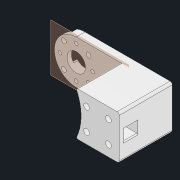
# Autodesk Inventor part: scara-base22
Saved by Autodesk Inventor 2022 (Build 260153000, 153)
## iProperties
Created: 2021-10-15
Part Number: scara-base22
Material: ABS プラスチック
Document SubType Name: Modeling
Designer: Yuta Kage
Density: 1.06 g/cm^3
Appearance: 滑らか - 白
Description: 印刷
Mass: 77.8231 g
Surface Area: 222.944 cm^2
Volume: 73.418 cm^3
Author: Yuta Kage
Autodesk Inventor part; units mm, degrees
ref_plane "YZ Plane" through (0, 0, 0) normal (1, 0, 0) x (0, 1, 0)
sketch "スケッチ1" plane through (0, 0, 0) normal (0, 0, 1) x (1, 0, 0)
  line L0 (0, -20) -> (80, -20)
  line L1 (80, -20) -> (80, 20)
  line L2 (80, 20) -> (0, 20)
  arc A0 (0, 20) -> (0, -20) centre (0, 0) ccw
  dimension "d0" = 40
  dimension "d2" = 40
  dimension "d51" = 80
  constraints: 6 end point, 2 point on circle, 1 centre point, 1 coincident, 1 horizontal, 1 parallel, 1 perpendicular
  measures "d0" distance of L0.end L1.end
  measures "d2" diameter of A0
  measures "d51" distance of L1.end L2.end
extrude "押し出し1" add sketch "スケッチ1" along normal blind 8
sketch "スケッチ2" plane through (0, 0, 8) normal (0, 0, 1) x (1, 0, 0)
  circle A0 centre (0, 0) radius 45
  line L0 (80, -20) -> (80, 20) projected
  line L1 (80, 20) -> (0, 20) projected
  line L2 (0, -20) -> (80, -20) projected
  arc A1 (0, 20) -> (0, -20) centre (0, 0) ccw projected
  point P0 (40.3113, 20)
  point P1 (40.3113, -20)
  point P2 (-40.3113, -20)
  point P3 (-40.3113, 20)
  dimension "d7" = 90
  constraints: 1 centre point, 1 coincident
  measures "d7" diameter of A0
extrude "押し出し2" add sketch "スケッチ2" along normal blind 40.5 contours A0 L1 L0 L2
sketch "スケッチ3" plane through (0, 0, 0) normal (0, 0, -1) x (-1, 0, 0)
  line L0 (-50, 10) -> (-70, 10)
  line L1 (-70, 10) -> (-70, -10)
  line L2 (-70, -10) -> (-50, -10)
  line L3 (-50, -10) -> (-50, 10)
  line L4 (-50, 10) -> (-70, -10) construction
  line L5 (-70, 10) -> (-50, -10) construction
  line L6 (-80, -20) -> (-80, 20) projected
  point P0 (-60, 0)
  point P1 (0, 0)
  dimension "d11" = 20
  dimension "d52" = 20
  dimension "d53" = 10
  constraints: 12 end point, 2 parallel, 1 horizontal, 1 horizontal alignment, 1 midpoint, 1 perpendicular
  measures "d11" distance of L1.end L0.end
  measures "d52" distance of L1.end L2.end
  measures "d53" distance between parallel lines of L6 L1
hole "穴1" at (50, -10, 0) at (50, 10, 0) at (70, -10, 0) at (70, 10, 0) direction (0, 0, 1) diameter 5.3 end through all clearance for "Socket Head Cap Screw" size "M5" standard "Ansi Metric M Profile"
sketch "スケッチ4" plane through (0, 0, 0) normal (0, 0, -1) x (-1, 0, 0)
  circle A0 centre (0, 0) radius 8.5
  dimension "d19" = 17
  constraints: 1 centre point, 1 coincident
  measures "d19" diameter of A0
extrude "押し出し3" cut sketch "スケッチ4" against normal blind 20
sketch "スケッチ5" plane through (0, 0, 0) normal (0, 0, -1) x (-1, 0, 0)
  circle A0 centre (0, 0) radius 15
  point P0 (0, -15)
  point P1 (15, 0)
  point P2 (0, 15)
  point P3 (-15, 0)
  dimension "d22" = 30
  dimension "d25" = 360
  constraints: 1 coincident, 1 vertical alignment, 7 other
hole "穴2" at (-15, 0, 0) at (0, 15, 0) at (0, -15, 0) at (15, 0, 0) direction (0, 0, 1) diameter 3.4 end through all clearance for "Socket Head Cap Screw" size "M3" standard "Ansi Metric M Profile"
sketch "スケッチ6" plane through (0, 0, 0) normal (0, 0, -1) x (-1, 0, 0)
  circle A0 centre (0, 0) radius 16
  point P0 (11.3137, -11.3137)
  point P1 (11.3137, 11.3137)
  point P2 (-11.3137, 11.3137)
  point P3 (-11.3137, -11.3137)
  dimension "d34" = 32
  dimension "d37" = 360
  constraints: 1 coincident, 1 horizontal alignment, 8 other
hole "穴3" at (-11.3137, -11.3137, 0) at (-11.3137, 11.3137, 0) at (11.3137, 11.3137, 0) at (11.3137, -11.3137, 0) direction (0, 0, 1) diameter 4.5 end through all counterbore diameter 8 counterbore depth 4 clearance for "Socket Head Cap Screw" size "M4" standard "Ansi Metric M Profile"
fillet "フィレット2" radius 2 2 edges at (80, -20, 24.25) (80, 20, 24.25)
fillet "フィレット5" radius 1 2 edges at (40.3113, 20, 28.25) (40.3113, -20, 28.25)
ref_plane "作業平面1" through (0, 0, 44.5) normal (0, 0, 1) x (1, 0, 0)
sketch "スケッチ7" plane through (0, 0, 44.5) normal (0, 0, 1) x (1, 0, 0)
  circle A0 centre (50, -10) radius 2.65 projected
  circle A1 centre (50, 10) radius 2.65 projected
  circle A2 centre (50, 10) radius 8
  circle A3 centre (50, -10) radius 2.65 projected
  circle A4 centre (50, -10) radius 9
  line L0 (43.755, -5) -> (80, -5)
  line L1 (80, -5) -> (80, 5)
  line L2 (80, 5) -> (43.755, 5)
  line L3 (43.755, 5) -> (43.755, -5)
  line L4 (43.755, -5) -> (80, 5) construction
  line L5 (80, -5) -> (43.755, 5) construction
  line L6 (80, -18) -> (80, 18) projected
  point P0 (0, 0)
  point P1 (61.8775, 0)
  point P2 (61.8775, 0)
  point P3 (43.755, -3.5193)
  point P4 (57.4833, -5)
  point P5 (56.245, 5)
  dimension "d59" = 16
  dimension "d64" = 18
  dimension "d65" = 10
  constraints: 12 end point, 3 midpoint, 2 coincident, 2 parallel, 1 centre point, 1 horizontal, 1 horizontal alignment, 1 perpendicular, 1 point on line, 3 other
  measures "d64" diameter of A4
  measures "d65" distance of L0.end L1.end
extrude "押し出し4" cut sketch "スケッチ7" against normal blind 13 contours A0 | A1 | A2 L2 | L2 A2 | A2 L2 L1 L0 A4 L3 | L3 L0 A4 | A4 L0 L3
sketch "スケッチ8" plane through (0, 0, 31.5) normal (0, 0, 1) x (1, 0, 0)
  circle A0 centre (50, 10) radius 5
  circle A1 centre (50, -10) radius 5
  circle A2 centre (50, -10) radius 2.65 projected
  circle A3 centre (50, 10) radius 2.65 projected
  point P0 (0, 0)
  dimension "d66" = 10
  dimension "d67" = 10
  constraints: 2 centre point, 2 coincident
  measures "d66" diameter of A0
  measures "d67" diameter of A1
extrude "押し出し5" add sketch "スケッチ8" along normal blind 0.5
sketch "スケッチ9" plane through (50, 10, 32) normal (0, 0, 1) x (1, 0, 0)
  circle A0 centre (0, -20) radius 5 projected
  circle A1 centre (0, 0) radius 5 projected
  circle A2 centre (0, -20) radius 3.95
  circle A3 centre (0, 0) radius 3.95
  circle A4 centre (0, -20) radius 2.65 projected
  circle A5 centre (0, 0) radius 2.65 projected
  point P0 (-50, -10)
  dimension "d70" = 7.9
  dimension "d71" = 7.9
  constraints: 2 centre point, 2 coincident
  measures "d70" diameter of A2
  measures "d71" diameter of A3
extrude "押し出し6" add sketch "スケッチ9" along normal blind 12 contours A2 | A3
sketch "スケッチ10" plane through (0, 0, 0) normal (0, 0, -1) x (-1, 0, 0)
  line L0 (50.5488, -20) -> (8, -20)
  line L1 (8, -20) -> (8, 20)
  line L2 (8, 20) -> (50.5488, 20)
  line L3 (50.5488, 20) -> (50.5488, -20)
  line L4 (50.5488, -20) -> (8, 20) construction
  line L5 (8, -20) -> (50.5488, 20) construction
  arc A0 (0, -20) -> (14.1421, -14.1421) centre (0, 0) ccw projected
  point P0 (29.2744, 0)
  point P1 (29.2744, 0)
  dimension "d75" = 8
  constraints: 12 end point, 3 midpoint, 2 parallel, 1 horizontal, 1 horizontal alignment, 1 perpendicular, 1 tangent
  measures "d75" distance from line of point (0, 0) L1
extrude "押し出し7" cut sketch "スケッチ10" against normal blind 4
fillet "フィレット6" radius 1 4 edges at (-8, 2.8723, 2) (-8, -2.8723, 2) (-8, 18.3303, 2) (-8, -18.3303, 2)
sketch "スケッチ11" plane through (0, 0, 44.5) normal (0, 0, -1) x (-1, 0, 0)
  circle A0 centre (-50, 10) radius 5 projected
  circle A1 centre (-50, -10) radius 5 projected
  circle A2 centre (-50, -10) radius 2.65 projected
  circle A3 centre (-50, 10) radius 2.65 projected
  point P0 (0, 0)
extrude "押し出し8" add sketch "スケッチ11" along normal blind 0.5
fillet "フィレット7" radius 1 6 edges at (57.4833, -5, 38) (42.4578, -14.9108, 38) (56.245, 5, 38) (42.8803, 13.6483, 38) (80, 5, 38) (80, -5, 38)
ref_plane "作業平面2" through (0, 0, 38) normal (0, 0, -1) x (-1, 0, 0)
sketch "スケッチ12" plane through (0, 0, 0) normal (0, 0, -1) x (-1, 0, 0)
  line L0 (5.5, 9) -> (-5.5, 9)
  line L1 (-5.5, 9) -> (-5.5, -9)
  line L2 (-5.5, -9) -> (5.5, -9)
  line L3 (5.5, -9) -> (5.5, 9)
  line L4 (5.5, 9) -> (-5.5, -9) construction
  line L5 (-5.5, 9) -> (5.5, -9) construction
  point P0 (0, 0)
  dimension "d84" = 11
  dimension "d85" = 18
  constraints: 12 end point, 2 midpoint, 2 parallel, 1 horizontal, 1 perpendicular
  measures "d84" distance of L2.end L1.end
  measures "d85" distance of L1.end L0.end
hole "穴4" at (-5.5, -9, 0) at (5.5, -9, 0) at (5.5, 9, 0) at (-5.5, 9, 0) direction (0, 0, 1) diameter 3.3 depth 4 tip angle 118
sketch "スケッチ13" plane through (0, 0, 0) normal (0, 0, -1) x (-1, 0, 0)
  circle A0 centre (-50, 10) radius 2.65 projected
  circle A1 centre (-50, -10) radius 2.65 projected
  circle A2 centre (-70, 10) radius 2.65 projected
  circle A3 centre (-70, -10) radius 2.65 projected
  circle A4 centre (-50, 10) radius 5
  circle A5 centre (-50, -10) radius 2.65 projected
  circle A6 centre (-50, -10) radius 5
  circle A7 centre (-70, 10) radius 5
  circle A8 centre (-70, -10) radius 5
  point P0 (0, 0)
  dimension "d93" = 10
  dimension "d94" = 10
  dimension "d95" = 10
  dimension "d96" = 10
  constraints: 4 centre point, 4 coincident
  measures "d93" diameter of A4
  measures "d94" diameter of A6
  measures "d95" diameter of A7
  measures "d96" diameter of A8
extrude "押し出し9" add sketch "スケッチ13" along normal blind 1
chamfer "面取り2" distance 1 angle 45 4 edges at (75, -10, 0) (55, -10, 0) (55, 10, 0) (75, 10, 0)
ref_plane "作業平面3" through (50, -10, 38) normal (0, 0, -1) x (-1, 0, 0)
ref_plane "作業平面4" through (0, 0, 8) normal (0, 0, 1) x (1, 0, 0)
equation "\"d71\" = d70"
